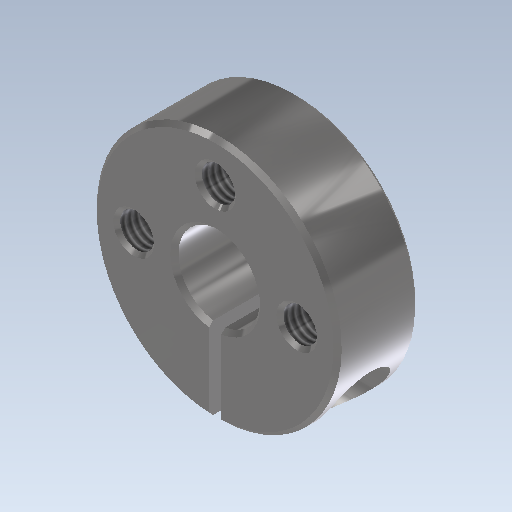
# Autodesk Inventor part: SCSTR10-10b
Saved by Autodesk Inventor 2021 (Build 250183000, 183)
## iProperties
Created: 2019-10-22
Part Number: SCSTR10-10b
Material: 鋼、炭素鋼
Catalog Web Link: www.cadenas.de
Description: SCST, PSCST, SSCST, SCSTR, PSCSTR, SSCSTR-b-Shaft Collars - 3 Holes/3 Taps
Vendor: MISUMI
Document SubType Name: Modeling
Designer: psadmin
Manufacturer: MISUMI
Mass: 41.0727 g
Surface Area: 31.3153 cm^2
Volume: 5.23219 cm^3
Density: 7.85 g/cm^3
Appearance: 半つや出し
Category: PARTsolutions
Company: MISUMI
PSOL_IDENT_0: {$CADENAS_DATA\23d-libs\misumi\metric\03_set_collars\scst\scst_b.prj},212 {VTYP=3D},{NB=SCSTR10-10b}
PSOL_IDENT_1: ,{LINA=SCSTR10-10},{NN=SCST, PSCST, SSCST, SCSTR, PSCSTR, SSCSTR-b},{DATE=30.03.2018 01:14:48},{GEOM
PSOL_IDENT_2: DATE=30.10.2015 01:43:51},{VERSION=},{LINEID=60},{WBVAR=TS,MAT,ST,BS},{WBNUMERIC=BS}  {NB=SCSTR10-10
PSOL_IDENT_3: b},{LINA=SCSTR10-10},{KT=DUMMY},{PN=SCSTR10-10},{TYPE=SCSTR},{TS=3T},{TSALG= '3H' , '3-Hole' , '3T'
PSOL_IDENT_4: , '3-Tapped' },{TSA='3H', '3-Hole', '3T', '3 Tap (Coarse)'},{MAT=S45C},{ST=BO},{STALG= 'BO' , 'Black
PSOL_IDENT_5: Oxide' , 'ENP' , 'Electroless Nickel Plating' },{AC=Hex Socket Head Cap Screw 1 pc.},{ACMAT=4137 Al
PSOL_IDENT_6: loy Steel},{D=10},{BS=10},{BALG= 8 , 10 },{D1=30},{M=M4},{M3D=4},{DD=4.5},{R=3.75},{W=1.5},{X=9.0},{
PSOL_IDENT_7: Y=5},{P=20},{C=0.5},{S=0.0},{M1=M5},{M13D=5},{L=15}
NN: SCST, PSCST, SSCST, SCSTR, PSCSTR, SSCSTR-b
NT: Shaft Collars - 3 Holes/3 Taps
NB: SCSTR10-10b
NBSYN: $PN.b
LINA: SCSTR10-10
PN: SCSTR10-10
TS: 3-Tapped
MAT: 1045 Carbon Steel
ST: Black Oxide
AC: Hex Socket Head Cap Screw 1 pc.
ACMAT: 4137 Alloy Steel
D: 10
BS: 10
D1: 30
M: M4
DD: 4.5
R: 3.75
W: 1.5
X: 9
Y: 5
P: 20
C: 0.5
S: 0
M1: M5
SUPPLIER: MISUMI
ARTICLENO: SCSTR10-10b
BOMINFO: SCSTR10-10
CREATOR: CADENAS GmbH
d17: 0.000 mm
Title: SCSTR10-10
Author: Cadenas PARTsolutions
Comments: Shaft Collars - 3 Holes/3 Taps
Autodesk Inventor part; units mm, degrees
sketch "Sketch_14" plane through (0, 0, 0) normal (1, 0, 0) x (0, 1, 0)
  line L0 (0, -5) -> (0, 5)
  line L1 (0, 5) -> (14.5, 5)
  line L2 (14.5, 5) -> (15, 4.5)
  line L3 (15, 4.5) -> (15, -4.5)
  line L4 (15, -4.5) -> (14.5, -5)
  line L5 (14.5, -5) -> (0, -5)
  line L6 (0, -5) -> (0, 5)
  constraints: 14 end point
revolve "Revolution1" add sketch "Sketch_14" angle 360 about axis through (0, 0, -5) along (0, 0, -1)
sketch "Sketch_15" plane through (0, 0, 0) normal (1, 0, 0) x (0, 1, 0)
  line L0 (0, -5) -> (0, 5)
  line L1 (0, 5) -> (5.5, 5)
  line L2 (5.5, 5) -> (5, 4.5)
  line L3 (5, 4.5) -> (5, -4.5)
  line L4 (5, -4.5) -> (5.5, -5)
  line L5 (5.5, -5) -> (0, -5)
  line L6 (0, -5) -> (0, 5)
  constraints: 14 end point
revolve "Revolution2" cut sketch "Sketch_15" angle 360 about axis through (0, 0, -5) along (0, 0, -1)
sketch "Sketch_16" plane through (0, 0, 0) normal (0, 0, 1) x (1, 0, 0)
  arc A0 (-0.75, -15.9824) -> (0.75, -15.9824) centre (0, 0) ccw
  line L0 (0.75, -15.9824) -> (0.75, 0)
  line L1 (0.75, 0) -> (-0.75, 0)
  line L2 (-0.75, 0) -> (-0.75, -15.9824)
  constraints: 6 end point, 2 point on circle, 1 centre point
extrude "Extrusion1" cut sketch "Sketch_16" along normal mid plane 10
sketch "Sketch_18" plane through (10, 0, 0) normal (1, 0, 0) x (0, 0, -1)
  line L0 (5, 0) -> (-5, 0)
  line L1 (-5, 0) -> (-5, 2.5)
  line L2 (-5, 2.5) -> (-4.567, 2.067)
  line L3 (-4.567, 2.067) -> (4.567, 2.067)
  line L4 (4.567, 2.067) -> (5, 2.5)
  line L5 (5, 2.5) -> (5, 0)
  line L6 (5, 0) -> (-5, 0)
  constraints: 14 end point
revolve "Revolution3" cut sketch "Sketch_18" angle 360 about axis through (10, 0, -5) along (0, 0, -1)
thread "Thread1" size "M5x0.8" class "6H" standard "ISO Metric profile" full length
sketch "Sketch_20" plane through (-10, 0, 0) normal (1, 0, 0) x (0, 0, -1)
  line L0 (5, 0) -> (-5, 0)
  line L1 (-5, 0) -> (-5, 2.5)
  line L2 (-5, 2.5) -> (-4.567, 2.067)
  line L3 (-4.567, 2.067) -> (4.567, 2.067)
  line L4 (4.567, 2.067) -> (5, 2.5)
  line L5 (5, 2.5) -> (5, 0)
  line L6 (5, 0) -> (-5, 0)
  constraints: 14 end point
revolve "Revolution4" cut sketch "Sketch_20" angle 360 about axis through (-10, 0, -5) along (0, 0, -1)
thread "Thread2" size "M5x0.8" class "6H" standard "ISO Metric profile" full length
sketch "Sketch_22" plane through (0, 10, 0) normal (0, 1, 0) x (1, 0, 0)
  line L0 (0, 5) -> (0, -5)
  line L1 (0, -5) -> (-2.5, -5)
  line L2 (-2.5, -5) -> (-2.067, -4.567)
  line L3 (-2.067, -4.567) -> (-2.067, 4.567)
  line L4 (-2.067, 4.567) -> (-2.5, 5)
  line L5 (-2.5, 5) -> (0, 5)
  line L6 (0, 5) -> (0, -5)
  constraints: 14 end point
revolve "Revolution5" cut sketch "Sketch_22" angle 360 about axis through (0, 10, -5) along (0, 0, -1)
thread "Thread3" size "M5x0.8" class "6H" standard "ISO Metric profile" full length
sketch "Sketch_23" plane through (0, -9, 0) normal (0, 1, 0) x (1, 0, 0)
  line L0 (15, 0) -> (0, 0)
  line L1 (0, 0) -> (0, 2.25)
  line L2 (0, 2.25) -> (5, 2.25)
  line L3 (5, 2.25) -> (5, 3.75)
  line L4 (5, 3.75) -> (15, 3.75)
  line L5 (15, 3.75) -> (15, 0)
  line L6 (15, 0) -> (0, 0)
  constraints: 14 end point
revolve "Revolution6" cut sketch "Sketch_23" angle 360 about axis through (15, -9, 0) along (1, 0, 0)
sketch "Sketch_25" plane through (0, 0, 0) normal (0, 0, 1) x (1, 0, 0)
  line L0 (-0.75, -9) -> (-13.2665, -9)
  line L1 (-13.2665, -9) -> (-13.2665, -7.379)
  line L2 (-13.2665, -7.379) -> (-1.129, -7.379)
  line L3 (-1.129, -7.379) -> (-0.75, -7)
  line L4 (-0.75, -7) -> (-0.75, -9)
  line L5 (-0.75, -9) -> (-13.2665, -9)
  constraints: 12 end point
revolve "Revolution7" cut sketch "Sketch_25" angle 360 about axis through (-0.75, -9, 0) along (1, 0, 0)
thread "Thread4" size "M4x0.7" class "6H" standard "ISO Metric profile" length 12.1375
ref_plane "to_bolt_XY" through (5, -9, 0) normal (1, 0, 0) x (0, 0, -1)
ref_plane "to_bolt_YZ" through (5, -9, 0) normal (0, 0, -1) x (0, 1, 0)
ref_plane "to_bolt_ZX" through (5, -9, 0) normal (0, 1, 0) x (1, 0, 0)
body "Solid1"
